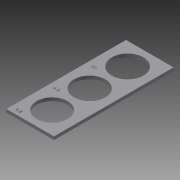
# Autodesk Inventor part: micGauge
Saved by Autodesk Inventor 2015 (Build 190159000, 159)
## iProperties
Created: 2015-12-14
Part Number: micGauge
Material: Generic
Document SubType Name: Modeling
Designer: mca20
Density: 1 g/cm^3
Appearance: Default
Author: mca20
Autodesk Inventor part; units mm, degrees
ref_plane "YZ Plane" through (0, 0, 0) normal (1, 0, 0) x (0, 1, 0)
ref_plane "XZ Plane" through (0, 0, 0) normal (0, 1, 0) x (-1, 0, 0)
ref_plane "XY Plane" through (0, 0, 0) normal (0, 0, 1) x (1, 0, 0)
sketch "Sketch2" plane through (0, 0, 0) normal (0, 1, 0) x (-1, 0, 0)
  line L0 (0, 0) -> (-15, 0)
  line L1 (-15, 0) -> (-15, -37.7)
  line L2 (-15, -37.7) -> (0, -37.7)
  line L3 (0, -37.7) -> (0, 0)
  dimension "d0" = 37.7
  dimension "d1" = 15
  constraints: 8 end point, 2 parallel, 1 horizontal, 1 perpendicular
  measures "d0" distance between parallel lines of L2 L0
  measures "d1" distance between parallel lines of L1 L3
extrude "Extrusion1" add sketch "Sketch2" along normal blind 1
sketch "Sketch4" plane through (0, 1, 0) normal (0, 1, 0) x (1, 0, 0)
  circle A0 centre (7.5, 6.9) radius 4.9
  line L0 (0, 37.7) -> (0, 0) projected
  line L1 (0, 0) -> (15, 0) projected
  circle A1 centre (7.5, 18.75) radius 4.95
  circle A2 centre (7.5, 30.7) radius 5
  dimension "d7" = 9.8
  dimension "d8" = 7.5
  dimension "d9" = 6.9
  dimension "d10" = 9.9
  dimension "d11" = 7.5
  dimension "d12" = 11.85
  dimension "d13" = 10
  dimension "d14" = 7.5
  dimension "d15" = 11.95
  dimension "d16" = 2
  dimension "d17" = 2
  dimension "d18" = 2
  constraints: 3 centre point
  measures "d7" diameter of A0
  measures "d8" distance from line of L0 A0.centre
  measures "d9" distance from line of L1 A0.centre
  measures "d10" diameter of A1
  measures "d11" distance from line of L0 A1.centre
  measures "d12" distance of A1.centre A0.centre
  measures "d13" diameter of A2
  measures "d14" distance from line of L0 A2.centre
  measures "d15" distance of A2.centre A1.centre
  measures "d18" distance edge to line of A0 L1
sketch "Sketch5" plane through (0, 1, 0) normal (0, 1, 0) x (1, 0, 0)
  line L0 (1.5, 2) -> (3.4173, 2) construction
  line L1 (3.4173, 2) -> (3.4173, 0.5649) construction
  line L2 (3.4173, 0.5649) -> (1.5, 0.5649) construction
  line L3 (1.5, 0.5649) -> (1.5, 2) construction
  line L4 (1.5, 13.8) -> (3.4173, 13.8) construction
  line L5 (3.4173, 13.8) -> (3.4173, 12.1229) construction
  line L6 (3.4173, 12.1229) -> (1.5, 12.1229) construction
  line L7 (1.5, 12.1229) -> (1.5, 13.8) construction
  line L8 (1.5, 25.7) -> (3.0008, 25.7) construction
  line L9 (3.0008, 25.7) -> (3.0008, 23.8136) construction
  line L10 (3.0008, 23.8136) -> (1.5, 23.8136) construction
  line L11 (1.5, 23.8136) -> (1.5, 25.7) construction
  line L12 (0, 37.7) -> (0, 0) projected
  line L13 (7.5373, 2) -> (-1.4627, 2)
  line L14 (7.5373, 13.8) -> (-1.4627, 13.8)
  line L15 (7.5373, 25.7) -> (-1.4627, 25.7)
  line L16 (0, 0) -> (15, 0) projected
  spline S0 degree 2 poles (1.5454, 1.6524) (1.5454, 1.7293) (1.5956, 1.8574) (1.6394, 1.9036) knots 0 0 0 1 2 2 2
  spline S1 degree 2 poles (1.6394, 1.9036) (1.6807, 1.9481) (1.8015, 1.9976) (1.863, 1.9976) knots 0 0 0 1 2 2 2
  spline S2 degree 2 poles (1.863, 1.9976) (1.9319, 1.9976) (2.0438, 1.9514) (2.0851, 1.9076) knots 0 0 0 1 2 2 2
  spline S3 degree 2 poles (2.0851, 1.9076) (2.137, 1.8525) (2.1937, 1.6742) (2.1937, 1.5373) knots 0 0 0 1 2 2 2
  spline S4 degree 2 poles (2.1937, 1.5373) (2.1937, 1.4133) (2.1378, 1.1912) (2.0835, 1.1175) knots 0 0 0 1 2 2 2
  spline S5 degree 2 poles (2.0835, 1.1175) (2.0259, 1.0397) (1.8639, 0.9579) (1.7455, 0.9579) knots 0 0 0 1 2 2 2
  spline S6 degree 2 poles (1.7455, 0.9579) (1.7188, 0.9579) (1.658, 0.9635) (1.6321, 0.9716) knots 0 0 0 1 2 2 2
  line L17 (1.6321, 0.9716) -> (1.6321, 1.1005)
  line L18 (1.6321, 1.1005) -> (1.6386, 1.1005)
  spline S7 degree 2 poles (1.6386, 1.1005) (1.6556, 1.0908) (1.7269, 1.0737) (1.7634, 1.0737) knots 0 0 0 1 2 2 2
  spline S8 degree 2 poles (1.7634, 1.0737) (1.8947, 1.0737) (2.0446, 1.2472) (2.0551, 1.4076) knots 0 0 0 1 2 2 2
  spline S9 degree 2 poles (2.0551, 1.4076) (2.0016, 1.3712) (1.9044, 1.3379) (1.8468, 1.3379) knots 0 0 0 1 2 2 2
  spline S10 degree 2 poles (1.8468, 1.3379) (1.7917, 1.3379) (1.7002, 1.3622) (1.654, 1.3971) knots 0 0 0 1 2 2 2
  spline S11 degree 2 poles (1.654, 1.3971) (1.6005, 1.4384) (1.5454, 1.564) (1.5454, 1.6524) knots 0 0 0 1 2 2 2
  spline S12 degree 2 poles (2.0583, 1.5673) (2.0583, 1.6686) (2.0211, 1.7966) (1.9878, 1.8314) knots 0 0 0 1 2 2 2
  spline S13 degree 2 poles (1.9878, 1.8314) (1.9587, 1.8639) (1.8979, 1.8882) (1.8622, 1.8882) knots 0 0 0 1 2 2 2
  spline S14 degree 2 poles (1.8622, 1.8882) (1.7796, 1.8882) (1.6815, 1.7699) (1.6815, 1.658) knots 0 0 0 1 2 2 2
  spline S15 degree 2 poles (1.6815, 1.658) (1.6815, 1.5948) (1.7139, 1.513) (1.7496, 1.4838) knots 0 0 0 1 2 2 2
  spline S16 degree 2 poles (1.7496, 1.4838) (1.7755, 1.4627) (1.8395, 1.4489) (1.8768, 1.4489) knots 0 0 0 1 2 2 2
  spline S17 degree 2 poles (1.8768, 1.4489) (1.9198, 1.4489) (2.0186, 1.4789) (2.0559, 1.5041) knots 0 0 0 1 2 2 2
  spline S18 degree 2 poles (2.0559, 1.5041) (2.0567, 1.5138) (2.0583, 1.547) (2.0583, 1.5673) knots 0 0 0 1 2 2 2
  line L19 (2.5381, 0.9773) -> (2.3776, 0.9773)
  line L20 (2.3776, 0.9773) -> (2.3776, 1.1686)
  line L21 (2.3776, 1.1686) -> (2.5381, 1.1686)
  line L22 (2.5381, 1.1686) -> (2.5381, 0.9773)
  spline S19 degree 2 poles (3.0421, 0.9546) (2.9676, 0.9546) (2.8452, 0.9992) (2.8023, 1.0405) knots 0 0 0 1 2 2 2
  spline S20 degree 2 poles (2.8023, 1.0405) (2.7601, 1.081) (2.7164, 1.1912) (2.7164, 1.2536) knots 0 0 0 1 2 2 2
  spline S21 degree 2 poles (2.7164, 1.2536) (2.7164, 1.3347) (2.8031, 1.4708) (2.8857, 1.5113) knots 0 0 0 1 2 2 2
  line L23 (2.8857, 1.5113) -> (2.8857, 1.5154)
  spline S22 degree 2 poles (2.8857, 1.5154) (2.812, 1.5583) (2.7407, 1.6605) (2.7407, 1.7366) knots 0 0 0 1 2 2 2
  spline S23 degree 2 poles (2.7407, 1.7366) (2.7407, 1.8493) (2.9109, 2) (3.0421, 2) knots 0 0 0 1 2 2 2
  spline S24 degree 2 poles (3.0421, 2) (3.1783, 2) (3.3428, 1.8574) (3.3428, 1.7455) knots 0 0 0 1 2 2 2
  spline S25 degree 2 poles (3.3428, 1.7455) (3.3428, 1.6783) (3.2642, 1.547) (3.1904, 1.5097) knots 0 0 0 1 2 2 2
  line L24 (3.1904, 1.5097) -> (3.1904, 1.5057)
  spline S26 degree 2 poles (3.1904, 1.5057) (3.278, 1.4652) (3.3679, 1.3485) (3.3679, 1.2561) knots 0 0 0 1 2 2 2
  spline S27 degree 2 poles (3.3679, 1.2561) (3.3679, 1.128) (3.1815, 0.9546) (3.0421, 0.9546) knots 0 0 0 1 2 2 2
  spline S28 degree 2 poles (3.2301, 1.2431) (3.2301, 1.3047) (3.1815, 1.3776) (3.1126, 1.4149) knots 0 0 0 1 2 2 2
  spline S29 degree 2 poles (3.1126, 1.4149) (3.09, 1.4279) (3.0138, 1.4579) (2.966, 1.4773) knots 0 0 0 1 2 2 2
  spline S30 degree 2 poles (2.966, 1.4773) (2.9109, 1.4408) (2.8517, 1.3323) (2.8517, 1.2634) knots 0 0 0 1 2 2 2
  spline S31 degree 2 poles (2.8517, 1.2634) (2.8517, 1.1726) (2.9611, 1.0543) (3.0438, 1.0543) knots 0 0 0 1 2 2 2
  spline S32 degree 2 poles (3.0438, 1.0543) (3.128, 1.0543) (3.2301, 1.1556) (3.2301, 1.2431) knots 0 0 0 1 2 2 2
  spline S33 degree 2 poles (3.2115, 1.7439) (3.2115, 1.8112) (3.1216, 1.9011) (3.0413, 1.9011) knots 0 0 0 1 2 2 2
  spline S34 degree 2 poles (3.0413, 1.9011) (2.9684, 1.9011) (2.8752, 1.8209) (2.8752, 1.752) knots 0 0 0 1 2 2 2
  spline S35 degree 2 poles (2.8752, 1.752) (2.8752, 1.7026) (2.923, 1.6337) (2.9708, 1.6062) knots 0 0 0 1 2 2 2
  spline S36 degree 2 poles (2.9708, 1.6062) (2.9911, 1.5948) (3.077, 1.5551) (3.1118, 1.5438) knots 0 0 0 1 2 2 2
  spline S37 degree 2 poles (3.1118, 1.5438) (3.1702, 1.5883) (3.2115, 1.6831) (3.2115, 1.7439) knots 0 0 0 1 2 2 2
  spline S38 degree 2 poles (1.5454, 13.4548) (1.5454, 13.5318) (1.5956, 13.6598) (1.6394, 13.706) knots 0 0 0 1 2 2 2
  spline S39 degree 2 poles (1.6394, 13.706) (1.6807, 13.7506) (1.8015, 13.8) (1.863, 13.8) knots 0 0 0 1 2 2 2
  spline S40 degree 2 poles (1.863, 13.8) (1.9319, 13.8) (2.0438, 13.7538) (2.0851, 13.71) knots 0 0 0 1 2 2 2
  spline S41 degree 2 poles (2.0851, 13.71) (2.137, 13.6549) (2.1937, 13.4767) (2.1937, 13.3397) knots 0 0 0 1 2 2 2
  spline S42 degree 2 poles (2.1937, 13.3397) (2.1937, 13.2157) (2.1378, 12.9937) (2.0835, 12.9199) knots 0 0 0 1 2 2 2
  spline S43 degree 2 poles (2.0835, 12.9199) (2.0259, 12.8421) (1.8639, 12.7603) (1.7455, 12.7603) knots 0 0 0 1 2 2 2
  spline S44 degree 2 poles (1.7455, 12.7603) (1.7188, 12.7603) (1.658, 12.766) (1.6321, 12.7741) knots 0 0 0 1 2 2 2
  line L25 (1.6321, 12.7741) -> (1.6321, 12.9029)
  line L26 (1.6321, 12.9029) -> (1.6386, 12.9029)
  spline S45 degree 2 poles (1.6386, 12.9029) (1.6556, 12.8932) (1.7269, 12.8762) (1.7634, 12.8762) knots 0 0 0 1 2 2 2
  spline S46 degree 2 poles (1.7634, 12.8762) (1.8947, 12.8762) (2.0446, 13.0496) (2.0551, 13.21) knots 0 0 0 1 2 2 2
  spline S47 degree 2 poles (2.0551, 13.21) (2.0016, 13.1736) (1.9044, 13.1404) (1.8468, 13.1404) knots 0 0 0 1 2 2 2
  spline S48 degree 2 poles (1.8468, 13.1404) (1.7917, 13.1404) (1.7002, 13.1647) (1.654, 13.1995) knots 0 0 0 1 2 2 2
  spline S49 degree 2 poles (1.654, 13.1995) (1.6005, 13.2408) (1.5454, 13.3665) (1.5454, 13.4548) knots 0 0 0 1 2 2 2
  spline S50 degree 2 poles (2.0583, 13.3697) (2.0583, 13.471) (2.0211, 13.599) (1.9878, 13.6339) knots 0 0 0 1 2 2 2
  spline S51 degree 2 poles (1.9878, 13.6339) (1.9587, 13.6663) (1.8979, 13.6906) (1.8622, 13.6906) knots 0 0 0 1 2 2 2
  spline S52 degree 2 poles (1.8622, 13.6906) (1.7796, 13.6906) (1.6815, 13.5723) (1.6815, 13.4605) knots 0 0 0 1 2 2 2
  spline S53 degree 2 poles (1.6815, 13.4605) (1.6815, 13.3972) (1.7139, 13.3154) (1.7496, 13.2862) knots 0 0 0 1 2 2 2
  spline S54 degree 2 poles (1.7496, 13.2862) (1.7755, 13.2652) (1.8395, 13.2514) (1.8768, 13.2514) knots 0 0 0 1 2 2 2
  spline S55 degree 2 poles (1.8768, 13.2514) (1.9198, 13.2514) (2.0186, 13.2814) (2.0559, 13.3065) knots 0 0 0 1 2 2 2
  spline S56 degree 2 poles (2.0559, 13.3065) (2.0567, 13.3162) (2.0583, 13.3494) (2.0583, 13.3697) knots 0 0 0 1 2 2 2
  line L27 (2.5381, 12.7797) -> (2.3776, 12.7797)
  line L28 (2.3776, 12.7797) -> (2.3776, 12.971)
  line L29 (2.3776, 12.971) -> (2.5381, 12.971)
  line L30 (2.5381, 12.971) -> (2.5381, 12.7797)
  spline S57 degree 2 poles (2.7123, 13.4548) (2.7123, 13.5318) (2.7626, 13.6598) (2.8063, 13.706) knots 0 0 0 1 2 2 2
  spline S58 degree 2 poles (2.8063, 13.706) (2.8476, 13.7506) (2.9684, 13.8) (3.03, 13.8) knots 0 0 0 1 2 2 2
  spline S59 degree 2 poles (3.03, 13.8) (3.0989, 13.8) (3.2107, 13.7538) (3.252, 13.71) knots 0 0 0 1 2 2 2
  spline S60 degree 2 poles (3.252, 13.71) (3.3039, 13.6549) (3.3606, 13.4767) (3.3606, 13.3397) knots 0 0 0 1 2 2 2
  spline S61 degree 2 poles (3.3606, 13.3397) (3.3606, 13.2157) (3.3047, 12.9937) (3.2504, 12.9199) knots 0 0 0 1 2 2 2
  spline S62 degree 2 poles (3.2504, 12.9199) (3.1929, 12.8421) (3.0308, 12.7603) (2.9125, 12.7603) knots 0 0 0 1 2 2 2
  spline S63 degree 2 poles (2.9125, 12.7603) (2.8857, 12.7603) (2.825, 12.766) (2.799, 12.7741) knots 0 0 0 1 2 2 2
  line L31 (2.799, 12.7741) -> (2.799, 12.9029)
  line L32 (2.799, 12.9029) -> (2.8055, 12.9029)
  spline S64 degree 2 poles (2.8055, 12.9029) (2.8225, 12.8932) (2.8938, 12.8762) (2.9303, 12.8762) knots 0 0 0 1 2 2 2
  spline S65 degree 2 poles (2.9303, 12.8762) (3.0616, 12.8762) (3.2115, 13.0496) (3.222, 13.21) knots 0 0 0 1 2 2 2
  spline S66 degree 2 poles (3.222, 13.21) (3.1686, 13.1736) (3.0713, 13.1404) (3.0138, 13.1404) knots 0 0 0 1 2 2 2
  spline S67 degree 2 poles (3.0138, 13.1404) (2.9587, 13.1404) (2.8671, 13.1647) (2.8209, 13.1995) knots 0 0 0 1 2 2 2
  spline S68 degree 2 poles (2.8209, 13.1995) (2.7674, 13.2408) (2.7123, 13.3665) (2.7123, 13.4548) knots 0 0 0 1 2 2 2
  spline S69 degree 2 poles (3.2253, 13.3697) (3.2253, 13.471) (3.188, 13.599) (3.1548, 13.6339) knots 0 0 0 1 2 2 2
  spline S70 degree 2 poles (3.1548, 13.6339) (3.1256, 13.6663) (3.0648, 13.6906) (3.0292, 13.6906) knots 0 0 0 1 2 2 2
  spline S71 degree 2 poles (3.0292, 13.6906) (2.9465, 13.6906) (2.8485, 13.5723) (2.8485, 13.4605) knots 0 0 0 1 2 2 2
  spline S72 degree 2 poles (2.8485, 13.4605) (2.8485, 13.3972) (2.8809, 13.3154) (2.9165, 13.2862) knots 0 0 0 1 2 2 2
  spline S73 degree 2 poles (2.9165, 13.2862) (2.9425, 13.2652) (3.0065, 13.2514) (3.0438, 13.2514) knots 0 0 0 1 2 2 2
  spline S74 degree 2 poles (3.0438, 13.2514) (3.0867, 13.2514) (3.1856, 13.2814) (3.2229, 13.3065) knots 0 0 0 1 2 2 2
  spline S75 degree 2 poles (3.2229, 13.3065) (3.2237, 13.3162) (3.2253, 13.3494) (3.2253, 13.3697) knots 0 0 0 1 2 2 2
  line L33 (2.1394, 24.6797) -> (1.6515, 24.6797)
  line L34 (1.6515, 24.6797) -> (1.6515, 24.7818)
  line L35 (1.6515, 24.7818) -> (1.8331, 24.7818)
  line L36 (1.8331, 24.7818) -> (1.8331, 25.452)
  line L37 (1.8331, 25.452) -> (1.6515, 25.452)
  line L38 (1.6515, 25.452) -> (1.6515, 25.5436)
  spline S76 degree 2 poles (1.6515, 25.5436) (1.7545, 25.5436) (1.8517, 25.6019) (1.8582, 25.683) knots 0 0 0 1 2 2 2
  line L39 (1.8582, 25.683) -> (1.9619, 25.683)
  line L40 (1.9619, 25.683) -> (1.9619, 24.7818)
  line L41 (1.9619, 24.7818) -> (2.1394, 24.7818)
  line L42 (2.1394, 24.7818) -> (2.1394, 24.6797)
  spline S77 degree 2 poles (2.9457, 25.1797) (2.9457, 24.9107) (2.7893, 24.6587) (2.6264, 24.6587) knots 0 0 0 1 2 2 2
  spline S78 degree 2 poles (2.6264, 24.6587) (2.4611, 24.6587) (2.3063, 24.9156) (2.3063, 25.1789) knots 0 0 0 1 2 2 2
  spline S79 degree 2 poles (2.3063, 25.1789) (2.3063, 25.4496) (2.4627, 25.7) (2.6264, 25.7) knots 0 0 0 1 2 2 2
  spline S80 degree 2 poles (2.6264, 25.7) (2.7909, 25.7) (2.9457, 25.4407) (2.9457, 25.1797) knots 0 0 0 1 2 2 2
  spline S81 degree 2 poles (2.7739, 24.875) (2.7934, 24.9245) (2.8096, 25.0768) (2.8096, 25.1797) knots 0 0 0 1 2 2 2
  spline S82 degree 2 poles (2.8096, 25.1797) (2.8096, 25.2827) (2.7934, 25.4342) (2.7731, 25.4853) knots 0 0 0 1 2 2 2
  spline S83 degree 2 poles (2.7731, 25.4853) (2.7528, 25.5363) (2.6823, 25.589) (2.6264, 25.589) knots 0 0 0 1 2 2 2
  spline S84 degree 2 poles (2.6264, 25.589) (2.5705, 25.589) (2.4984, 25.5363) (2.4773, 25.4836) knots 0 0 0 1 2 2 2
  spline S85 degree 2 poles (2.4773, 25.4836) (2.4571, 25.4326) (2.4425, 25.277) (2.4425, 25.1789) knots 0 0 0 1 2 2 2
  spline S86 degree 2 poles (2.4425, 25.1789) (2.4425, 25.0736) (2.4554, 24.9326) (2.4765, 24.8775) knots 0 0 0 1 2 2 2
  spline S87 degree 2 poles (2.4765, 24.8775) (2.4959, 24.8256) (2.5681, 24.7697) (2.6264, 24.7697) knots 0 0 0 1 2 2 2
  spline S88 degree 2 poles (2.6264, 24.7697) (2.6815, 24.7697) (2.7536, 24.8224) (2.7739, 24.875) knots 0 0 0 1 2 2 2
  dimension "d19" = 1.9173
  dimension "d20" = 1.5
  dimension "d21" = 1.5
  dimension "d22" = 1.5
  dimension "d23" = 9
  dimension "d24" = 9
  dimension "d25" = 9
  dimension "d27" = 0
  dimension "d28" = 2
  dimension "d29" = 0
  dimension "d30" = 13.8
  dimension "d31" = 0
  dimension "d32" = 25.7
  constraints: 6 end point, 3 horizontal, 6 other
  measures "d19" distance of L0.start L0.end
  measures "d20" distance between parallel lines of L12 L3
  measures "d21" distance between parallel lines of L12 L7
  measures "d22" distance between parallel lines of L12 L11
  measures "d23" distance of L13.start L13.end
  measures "d24" distance of L14.start L14.end
  measures "d25" distance of L15.start L15.end
  measures "d27" distance between parallel lines of L13 L0
  measures "d28" distance between parallel lines of L16 L13
  measures "d29" distance between parallel lines of L14 L4
  measures "d30" distance between parallel lines of L16 L14
  measures "d31" distance between parallel lines of L8 L15
  measures "d32" distance between parallel lines of L16 L15
extrude "Extrusion2" cut sketch "Sketch5" against normal blind 0.5
extrude "Extrusion3" cut sketch "Sketch4" against normal blind 1
equation "\"d11\" = d8"
equation "\"d14\" = d8"
equation "\"d21\" = d20"
equation "\"d22\" = d20"
body "Solid1"
